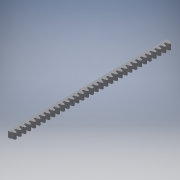
# Autodesk Inventor part: cremalheira
Saved by Autodesk Inventor 2018 (Build 220112000, 112)
## iProperties
Created: 2018-06-04
Part Number: cremalheira
Material: Genérico
Document SubType Name: Modeling
Designer: Ernandes
Density: 1 g/cm^3
Appearance: Padrão
Author: Ernandes
Autodesk Inventor part; units mm, degrees
ref_plane "YZ Plane" through (0, 0, 0) normal (1, 0, 0) x (0, 1, 0)
ref_plane "XZ Plane" through (0, 0, 0) normal (0, 1, 0) x (-1, 0, 0)
ref_plane "XY Plane" through (0, 0, 0) normal (0, 0, 1) x (1, 0, 0)
sketch "Esboço1" plane through (0, 0, 0) normal (0, 0, 1) x (1, 0, 0)
  line L0 (17.646, -58.134) -> (17.646, -57.09)
  line L1 (17.646, -57.09) -> (19.978, -56.658)
  line L2 (19.978, -56.658) -> (22.126, -55.788)
  line L3 (22.126, -55.788) -> (22.126, -54.192)
  line L4 (22.126, -54.192) -> (19.978, -53.324)
  line L5 (19.978, -53.324) -> (17.646, -52.892)
  line L6 (17.646, -50.802) -> (19.978, -50.37)
  line L7 (19.978, -50.37) -> (22.126, -49.5)
  line L8 (22.126, -49.5) -> (22.126, -47.904)
  line L9 (22.126, -47.904) -> (19.978, -47.036)
  line L10 (19.978, -47.036) -> (17.646, -46.604)
  line L11 (17.646, -44.514) -> (19.978, -44.082)
  line L12 (19.978, -44.082) -> (22.126, -43.212)
  line L13 (22.126, -43.212) -> (22.126, -41.616)
  line L14 (22.126, -41.616) -> (19.978, -40.748)
  line L15 (19.978, -40.748) -> (17.646, -40.316)
  line L16 (17.646, -38.226) -> (19.978, -37.794)
  line L17 (19.978, -37.794) -> (22.126, -36.924)
  line L18 (22.126, -36.924) -> (22.126, -35.328)
  line L19 (22.126, -35.328) -> (19.978, -34.46)
  line L20 (19.978, -34.46) -> (17.646, -34.028)
  line L21 (17.646, -31.938) -> (19.978, -31.506)
  line L22 (19.978, -31.506) -> (22.126, -30.636)
  line L23 (22.126, -30.636) -> (22.126, -29.04)
  line L24 (22.126, -29.04) -> (19.978, -28.172)
  line L25 (19.978, -28.172) -> (17.646, -27.74)
  line L26 (17.646, -25.65) -> (19.978, -25.218)
  line L27 (19.978, -25.218) -> (22.126, -24.348)
  line L28 (22.126, -24.348) -> (22.126, -22.752)
  line L29 (22.126, -22.752) -> (19.978, -21.884)
  line L30 (19.978, -21.884) -> (17.646, -21.452)
  line L31 (17.646, -19.362) -> (19.978, -18.93)
  line L32 (19.978, -18.93) -> (22.126, -18.06)
  line L33 (22.126, -18.06) -> (22.126, -16.464)
  line L34 (22.126, -16.464) -> (19.978, -15.596)
  line L35 (19.978, -15.596) -> (17.646, -15.164)
  line L36 (17.646, -13.074) -> (19.978, -12.642)
  line L37 (19.978, -12.642) -> (22.126, -11.7721)
  line L38 (22.126, -11.7721) -> (22.126, -10.176)
  line L39 (22.126, -10.176) -> (19.978, -9.308)
  line L40 (19.978, -9.308) -> (17.646, -8.876)
  line L41 (17.646, -6.7861) -> (19.978, -6.3541)
  line L42 (19.978, -6.3541) -> (22.126, -5.4841)
  line L43 (22.126, -5.4841) -> (22.126, -3.888)
  line L44 (22.126, -3.888) -> (19.978, -3.02)
  line L45 (19.978, -3.02) -> (17.646, -2.588)
  line L46 (17.646, -0.4981) -> (19.978, -0.0661)
  line L47 (19.978, -0.0661) -> (22.126, 0.8039)
  line L48 (22.126, 0.8039) -> (22.126, 2.3999)
  line L49 (22.126, 2.3999) -> (19.978, 3.268)
  line L50 (19.978, 3.268) -> (17.646, 3.6999)
  line L51 (17.646, 5.7899) -> (19.978, 6.2219)
  line L52 (19.978, 6.2219) -> (22.126, 7.0919)
  line L53 (22.126, 7.0919) -> (22.126, 8.6879)
  line L54 (22.126, 8.6879) -> (19.978, 9.5559)
  line L55 (19.978, 9.5559) -> (17.646, 9.9879)
  line L56 (17.646, 12.0779) -> (19.978, 12.5099)
  line L57 (19.978, 12.5099) -> (22.126, 13.3799)
  line L58 (22.126, 13.3799) -> (22.126, 14.9759)
  line L59 (22.126, 14.9759) -> (19.978, 15.8439)
  line L60 (19.978, 15.8439) -> (17.646, 16.2759)
  line L61 (17.646, 18.3659) -> (19.978, 18.7979)
  line L62 (19.978, 18.7979) -> (22.126, 19.6679)
  line L63 (22.126, 19.6679) -> (22.126, 21.2639)
  line L64 (22.126, 21.2639) -> (19.978, 22.1319)
  line L65 (19.978, 22.1319) -> (17.646, 22.5639)
  line L66 (17.646, 24.6539) -> (19.978, 25.0859)
  line L67 (19.978, 25.0859) -> (22.126, 25.9559)
  line L68 (22.126, 25.9559) -> (22.126, 27.5519)
  line L69 (22.126, 27.5519) -> (19.978, 28.4199)
  line L70 (19.978, 28.4199) -> (17.646, 28.8519)
  line L71 (17.646, 30.9419) -> (19.978, 31.3739)
  line L72 (19.978, 31.3739) -> (22.126, 32.2439)
  line L73 (22.126, 32.2439) -> (22.126, 33.8399)
  line L74 (22.126, 33.8399) -> (19.978, 34.7079)
  line L75 (19.978, 34.7079) -> (17.646, 35.1399)
  line L76 (17.646, 37.2299) -> (19.978, 37.6619)
  line L77 (19.978, 37.6619) -> (22.126, 38.5319)
  line L78 (22.126, 38.5319) -> (22.126, 40.1279)
  line L79 (22.126, 40.1279) -> (19.978, 40.9959)
  line L80 (19.978, 40.9959) -> (17.646, 41.4279)
  line L81 (17.646, 43.5179) -> (19.978, 43.9499)
  line L82 (19.978, 43.9499) -> (22.126, 44.8199)
  line L83 (22.126, 44.8199) -> (22.126, 46.4159)
  line L84 (22.126, 46.4159) -> (19.978, 47.2839)
  line L85 (19.978, 47.2839) -> (17.646, 47.7159)
  line L86 (17.646, 49.8059) -> (19.978, 50.2379)
  line L87 (19.978, 50.2379) -> (22.126, 51.1079)
  line L88 (22.126, 51.1079) -> (22.126, 52.7039)
  line L89 (22.126, 52.7039) -> (19.978, 53.5719)
  line L90 (19.978, 53.5719) -> (17.646, 54.0039)
  line L91 (17.646, 56.0939) -> (19.978, 56.5259)
  line L92 (19.978, 56.5259) -> (22.126, 57.3959)
  line L93 (22.126, 57.3959) -> (22.126, 58.9919)
  line L94 (22.126, 58.9919) -> (19.978, 59.8599)
  line L95 (19.978, 59.8599) -> (17.646, 60.2919)
  line L96 (17.646, 62.3818) -> (19.978, 62.8139)
  line L97 (19.978, 62.8139) -> (22.126, 63.6838)
  line L98 (22.126, 63.6838) -> (22.126, 65.2799)
  line L99 (22.126, 65.2799) -> (19.978, 66.1479)
  line L100 (19.978, 66.1479) -> (17.646, 66.5799)
  line L101 (17.646, 68.6698) -> (19.978, 69.1018)
  line L102 (19.978, 69.1018) -> (22.126, 69.9718)
  line L103 (22.126, 69.9718) -> (22.126, 71.5678)
  line L104 (22.126, 71.5678) -> (19.978, 72.4359)
  line L105 (19.978, 72.4359) -> (17.646, 72.8679)
  line L106 (17.646, 74.9578) -> (19.978, 75.3898)
  line L107 (19.978, 75.3898) -> (22.126, 76.2598)
  line L108 (22.126, 76.2598) -> (22.126, 77.8558)
  line L109 (22.126, 77.8558) -> (19.978, 78.7238)
  line L110 (19.978, 78.7238) -> (17.646, 79.1558)
  line L111 (17.646, 81.2458) -> (19.978, 81.6778)
  line L112 (19.978, 81.6778) -> (22.126, 82.5478)
  line L113 (22.126, 82.5478) -> (22.126, 84.1438)
  line L114 (22.126, 84.1438) -> (19.978, 85.0118)
  line L115 (19.978, 85.0118) -> (17.646, 85.4438)
  line L116 (17.646, 87.5338) -> (19.978, 87.9658)
  line L117 (19.978, 87.9658) -> (22.126, 88.8358)
  line L118 (22.126, 88.8358) -> (22.126, 90.4318)
  line L119 (22.126, 90.4318) -> (19.978, 91.2998)
  line L120 (19.978, 91.2998) -> (17.646, 91.7318)
  line L121 (17.646, 93.8218) -> (19.978, 94.2538)
  line L122 (19.978, 94.2538) -> (22.126, 95.1238)
  line L123 (22.126, 95.1238) -> (22.126, 96.7198)
  line L124 (22.126, 96.7198) -> (19.978, 97.5878)
  line L125 (19.978, 97.5878) -> (17.646, 98.0198)
  line L126 (17.646, 100.1098) -> (19.978, 100.5418)
  line L127 (19.978, 100.5418) -> (22.126, 101.4118)
  line L128 (22.126, 101.4118) -> (22.126, 103.0078)
  line L129 (22.126, 103.0078) -> (19.978, 103.8758)
  line L130 (19.978, 103.8758) -> (17.646, 104.3078)
  line L131 (17.646, 106.3978) -> (19.978, 106.8298)
  line L132 (19.978, 106.8298) -> (22.126, 107.6998)
  line L133 (22.126, 107.6998) -> (22.126, 109.2958)
  line L134 (22.126, 109.2958) -> (19.978, 110.1638)
  line L135 (19.978, 110.1638) -> (17.646, 110.5958)
  line L136 (17.646, 112.6858) -> (19.978, 113.1178)
  line L137 (19.978, 113.1178) -> (22.126, 113.9878)
  line L138 (22.126, 113.9878) -> (22.126, 115.5838)
  line L139 (22.126, 115.5838) -> (19.978, 116.4518)
  line L140 (19.978, 116.4518) -> (17.646, 116.8838)
  line L141 (17.646, 118.9738) -> (19.978, 119.4058)
  line L142 (19.978, 119.4058) -> (22.126, 120.2758)
  line L143 (22.126, 120.2758) -> (22.126, 121.8718)
  line L144 (22.126, 121.8718) -> (19.978, 122.7398)
  line L145 (19.978, 122.7398) -> (17.646, 123.1718)
  line L146 (17.646, 125.2618) -> (19.978, 125.6938)
  line L147 (19.978, 125.6938) -> (22.126, 126.5638)
  line L148 (22.126, 126.5638) -> (22.126, 128.1598)
  line L149 (22.126, 128.1598) -> (19.978, 129.0278)
  line L150 (19.978, 129.0278) -> (17.646, 129.4598)
  line L151 (17.646, 131.5498) -> (19.978, 131.9818)
  line L152 (19.978, 131.9818) -> (22.126, 132.8518)
  line L153 (22.126, 132.8518) -> (22.126, 134.4478)
  line L154 (22.126, 134.4478) -> (19.978, 135.3158)
  line L155 (19.978, 135.3158) -> (17.646, 135.7478)
  line L156 (17.646, 137.8377) -> (19.978, 138.2698)
  line L157 (19.978, 138.2698) -> (22.126, 139.1397)
  line L158 (22.126, 139.1397) -> (22.126, 140.7358)
  line L159 (22.126, 140.7358) -> (19.978, 141.6038)
  line L160 (19.978, 141.6038) -> (17.646, 142.0358)
  line L161 (17.646, 144.1257) -> (19.978, 144.5577)
  line L162 (19.978, 144.5577) -> (22.126, 145.4277)
  line L163 (22.126, 145.4277) -> (22.126, 147.0237)
  line L164 (22.126, 147.0237) -> (19.978, 147.8918)
  line L165 (19.978, 147.8918) -> (17.646, 148.3238)
  line L166 (17.646, -58.134) -> (14.646, -58.134)
  line L167 (14.646, -58.134) -> (14.646, 106.0305)
  line L168 (14.646, 106.0305) -> (14.646, 148.1078)
  line L169 (17.646, 148.3238) -> (14.646, 148.3238)
  line L170 (14.646, 148.3238) -> (14.646, 148.1078)
  line L171 (17.646, 142.0358) -> (17.646, 144.1257)
  line L172 (17.646, 125.2618) -> (17.646, 123.1718)
  line L173 (17.646, 118.9738) -> (17.646, 116.8838)
  line L174 (17.646, 112.6858) -> (17.646, 110.5958)
  line L175 (17.646, 106.3978) -> (17.646, 104.3078)
  line L176 (17.646, 100.1098) -> (17.646, 98.0198)
  line L177 (17.646, 93.8218) -> (17.646, 91.7318)
  line L178 (17.646, 87.5338) -> (17.646, 85.4438)
  line L179 (17.646, 81.2458) -> (17.646, 79.1558)
  line L180 (17.646, 74.9578) -> (17.646, 72.8679)
  line L181 (17.646, 68.6698) -> (17.646, 66.5799)
  line L182 (17.646, 62.3818) -> (17.646, 60.2919)
  line L183 (17.646, 56.0939) -> (17.646, 54.0039)
  line L184 (17.646, 49.8059) -> (17.646, 47.7159)
  line L185 (17.646, 43.5179) -> (17.646, 41.4279)
  line L186 (17.646, 37.2299) -> (17.646, 35.1399)
  line L187 (17.646, 30.9419) -> (17.646, 28.8519)
  line L188 (17.646, 24.6539) -> (17.646, 22.5639)
  line L189 (17.646, 18.3659) -> (17.646, 16.2759)
  line L190 (17.646, 12.0779) -> (17.646, 9.9879)
  line L191 (17.646, 5.7899) -> (17.646, 3.6999)
  line L192 (17.646, -0.4981) -> (17.646, -2.588)
  line L193 (17.646, -6.7861) -> (17.646, -8.876)
  line L194 (17.646, -13.074) -> (17.646, -15.164)
  line L195 (17.646, -19.362) -> (17.646, -21.452)
  line L196 (17.646, -25.65) -> (17.646, -27.74)
  line L197 (17.646, -31.938) -> (17.646, -34.028)
  line L198 (17.646, -38.226) -> (17.646, -40.316)
  line L199 (17.646, -44.514) -> (17.646, -46.604)
  line L200 (17.646, -50.802) -> (17.646, -52.892)
  line L201 (17.646, 137.8377) -> (17.646, 135.7478)
  line L202 (17.646, 131.5498) -> (17.646, 129.4598)
  point P0 (0, 0)
  dimension "d0" = 3
  constraints: 406 end point, 27 collinear, 6 vertical, 2 horizontal, 2 perpendicular, 2 point on line, 1 parallel
  measures "d0" distance of L0.start L166.end
extrude "Extrusão1" add sketch "Esboço1" along normal blind 10
offset faces "Tamanho1" outward -2.5 faces at (15.646, 5.3195, 10)
